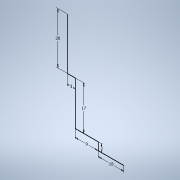
# Autodesk Inventor part: voorkant
Saved by Autodesk Inventor 2021 (Build 250183000, 183)
## iProperties
Created: 2022-02-01
Part Number: voorkant
Material: Generic
Document SubType Name: Modeling
Designer: ryan
Density: 1 g/cm^3
Appearance: Default
Author: ryan
Autodesk Inventor part; units mm, degrees
ref_plane "YZ Plane" through (0, 0, 0) normal (1, 0, 0) x (0, 1, 0)
ref_plane "XZ Plane" through (0, 0, 0) normal (0, 1, 0) x (-1, 0, 0)
ref_plane "XY Plane" through (0, 0, 0) normal (0, 0, 1) x (1, 0, 0)
sketch "Sketch1" plane through (0, 0, 0) normal (0, 0, 1) x (1, 0, 0)
  line L0 (0, 0) -> (0, -20)
  line L1 (0, -20) -> (3, -20)
  line L2 (3, -20) -> (3, -37)
  line L3 (3, -37) -> (13, -37)
  line L4 (13, -37) -> (13, -40)
  line L5 (13, -40) -> (25, -40)
  line L6 (25, -40) -> (25, -37)
  line L7 (25, -37) -> (35, -37)
  line L8 (0, 0) -> (3, 0)
  line L9 (3, 0) -> (3, 20)
  line L10 (3, 20) -> (0, 20)
  line L11 (0, 20) -> (0, 30)
  line L12 (0, 30) -> (3, 30)
  line L13 (3, 30) -> (35, 30)
  line L14 (35, 30) -> (35, -37)
  dimension "d0" = 20
  dimension "d1" = 3
  dimension "d2" = 17
  dimension "d3" = 10
  dimension "d4" = 3
  dimension "d5" = 12
  dimension "d6" = 3
  dimension "d7" = 10
  dimension "d8" = 3
  dimension "d9" = 20
  dimension "d10" = 3
  dimension "d11" = 10
  dimension "d12" = 3
  dimension "d13" = 32
  constraints: 30 end point, 8 perpendicular, 3 vertical, 2 horizontal, 1 point on line
  measures "d0" distance of L0.start L0.end
  measures "d1" distance of L0.end L1.end
  measures "d2" distance of L1.end L2.end
  measures "d3" distance of L2.end L3.end
  measures "d4" distance of L3.end L4.end
  measures "d5" distance of L4.end L5.end
  measures "d6" distance of L5.end L6.end
  measures "d7" distance of L6.end L7.end
  measures "d8" distance of L0.start L8.end
  measures "d9" distance of L8.end L9.end
  measures "d10" distance of L9.end L10.end
  measures "d11" distance of L10.end L11.end
  measures "d12" distance of L11.end L12.end
  measures "d13" distance of L12.end L13.end
extrude "Extrusion1" add sketch "Sketch1" along normal blind 3
mirror "Mirror1" about plane through (35, 30, 0) normal (0, 1, 0) of "Extrusion1"
body "Solid1"
